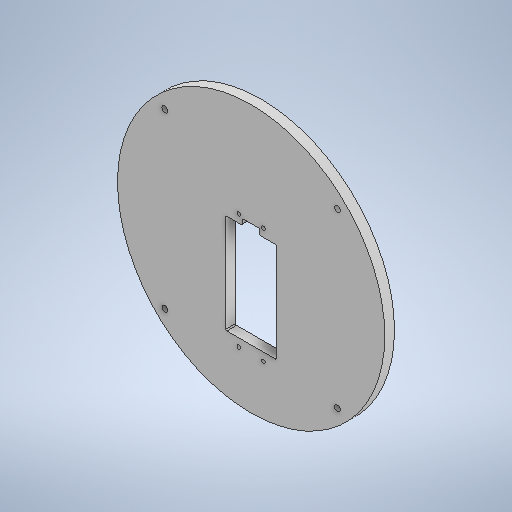
# Autodesk Inventor part: bottom-plate
Saved by Autodesk Inventor 2025 (Build 290162000, 162)
## iProperties
Created: 2024-05-28
Part Number: bottom-plate
Material: Generic
Document SubType Name: Modeling
Designer: hifzh
Density: 1 g/cm^3
Appearance: Default
Author: hifzh
## iProperties of the stored document bottom-plate_3DPrint.ipt
Created: 2024-07-12
Part Number: bottom-plate_3DPrint
Material: Generic
Document SubType Name: Modeling
Designer: hifzhil
Density: 1 g/cm^3
Appearance: Default
Author: hifzhil
Autodesk Inventor part; units mm, degrees
sketch "Sketch1" plane through (0, 0, 0) normal (0, 0, 1) x (1, 0, 0)
  circle A0 centre (0, 0) radius 55
  dimension "d0" = 110
  constraints: 1 centre point, 1 coincident
  measures "d0" diameter of A0
extrude "Extrusion1" add sketch "Sketch1" along normal blind 4
ref_plane "Work Plane1" through (0, 0, 4) normal (0, 0, 1) x (1, 0, 0)
sketch "Sketch2" plane through (0, 0, 4) normal (0, 0, 1) x (1, 0, 0)
  line L0 (-10.406, 10.152) -> (10.406, 10.152)
  line L1 (10.406, 10.152) -> (10.406, -30.726)
  line L2 (10.406, -30.726) -> (-10.406, -30.726)
  line L3 (-10.406, -30.726) -> (-10.406, 10.152)
  circle A0 centre (-35.532, 35.532) radius 1.5
  circle A1 centre (-35.532, -35.532) radius 1.5
  circle A2 centre (35.532, -35.532) radius 1.5
  circle A3 centre (35.532, 35.532) radius 1.5
  circle A4 centre (-5.08, 13.462) radius 1
  circle A5 centre (5.08, 13.462) radius 1
  circle A6 centre (-5.08, -34.036) radius 1
  circle A7 centre (5.08, -34.036) radius 1
  point P0 (0, 0)
  point P1 (0, 10.152)
  point P2 (0, -30.726)
  dimension "d78" = 30.226
  dimension "d80" = 5.08
  dimension "d82" = 5.08
  dimension "d4" = 20.812
  dimension "d5" = 40.878
  dimension "d6" = 10.152
  dimension "d7" = 3
  dimension "d8" = 3
  dimension "d9" = 3
  dimension "d10" = 3
  dimension "d11" = 2
  dimension "d12" = 2
  dimension "d13" = 2
  dimension "d14" = 2
  dimension "d15" = 35.532
  dimension "d16" = 35.532
  dimension "d17" = 35.532
  dimension "d18" = 35.532
  dimension "d19" = 35.532
  dimension "d20" = 35.532
  dimension "d21" = 35.532
  dimension "d22" = 35.532
  dimension "d23" = 10.16
  dimension "d24" = 10.16
  dimension "d25" = 3.31
  dimension "d26" = 3.31
  dimension "d27" = 3.31
  dimension "d28" = 3.31
  dimension "d47" = 30.726
  dimension "d48" = 5.08
  dimension "d49" = 5.08
  dimension "d50" = 5.08
  dimension "d51" = 5.08
  dimension "d137" = 10.152
  constraints: 8 centre point, 8 end point, 2 midpoint, 2 parallel, 1 horizontal, 1 perpendicular, 1 vertical alignment
  measures "d4" distance of L0.start L0.end
  measures "d5" distance of L0.end L1.end
  measures "d6" distance from line of point (0, 0) L0
  measures "d7" diameter of A0
  measures "d8" diameter of A1
  measures "d9" diameter of A2
  measures "d10" diameter of A3
  measures "d11" diameter of A4
  measures "d12" diameter of A5
  measures "d13" diameter of A6
  measures "d14" diameter of A7
  measures "d15" horizontal distance of point (0, 0) A0.centre
  measures "d16" horizontal distance of point (0, 0) A0.centre
  measures "d17" horizontal distance of point (0, 0) A3.centre
  measures "d18" horizontal distance of point (0, 0) A3.centre
  measures "d19" horizontal distance of point (0, 0) A2.centre
  measures "d20" horizontal distance of point (0, 0) A2.centre
  measures "d21" horizontal distance of point (0, 0) A1.centre
  measures "d22" horizontal distance of point (0, 0) A1.centre
  measures "d23" distance of A5.centre A4.centre
  measures "d24" distance of A7.centre A6.centre
  measures "d25" distance from line of L0 A4.centre
  measures "d26" distance from line of L0 A5.centre
  measures "d27" distance from line of L2 A6.centre
  measures "d28" distance from line of L2 A7.centre
  measures "d47" distance of point (0, -30.726) point (0, 0)
  measures "d48" horizontal distance of point (0, 0) A5.centre
  measures "d49" horizontal distance of point (0, 0) A4.centre
  measures "d50" horizontal distance of point (0, 0) A7.centre
  measures "d51" horizontal distance of point (0, 0) A6.centre
  measures "d137" distance of point (0, 10.152) point (0, 0)
extrude "Extrusion2" cut sketch "Sketch2" against normal blind 4 contours L0 L1 L2 L3
ref_plane "Work Plane2" through (0, 0, 4) normal (0, 0, 1) x (1, 0, 0)
sketch "Sketch3" plane through (0, 0, 4) normal (0, 0, 1) x (1, 0, 0)
  circle A0 centre (-35.577, 35.5342) radius 2.5
  circle A1 centre (-35.5225, -35.5931) radius 2.5
  circle A2 centre (35.5095, -35.5931) radius 2.5
  circle A3 centre (35.5095, 35.4262) radius 2.5
  point P0 (0, 0)
  constraints: 4 centre point
ref_plane "Work Plane3" through (0, 0, 0) normal (0, 0, 1) x (1, 0, 0)
sketch "Sketch4" plane through (0, 0, 0) normal (0, 0, 1) x (1, 0, 0)
  circle A0 centre (-35.577, 35.5342) radius 2.5
  circle A1 centre (-35.5225, -35.5931) radius 2.5
  circle A2 centre (35.5095, -35.5931) radius 2.5
  circle A3 centre (35.5095, 35.4262) radius 2.5
  point P0 (0, 0)
  point P1 (0, 0)
  dimension "d41" = 5
  dimension "d42" = 5
  dimension "d43" = 5
  dimension "d44" = 5
  constraints: 4 centre point
  measures "d41" diameter of A0
  measures "d42" diameter of A1
  measures "d43" diameter of A2
  measures "d44" diameter of A3
extrude "Extrusion3" cut sketch "Sketch4" along normal blind 0.657
ref_plane "Work Plane4" through (0, 0, 0) normal (0, 0, -1) x (-1, 0, 0)
sketch "Sketch5" plane through (0, 0, 0) normal (0, 0, -1) x (-1, 0, 0)
  line L0 (-9.906, 9.652) -> (9.906, 9.652)
  line L1 (9.906, 9.652) -> (9.906, -30.226)
  line L2 (9.906, -30.226) -> (-9.906, -30.226)
  line L3 (-9.906, -30.226) -> (-9.906, 9.652)
  circle A0 centre (-35.532, 35.532) radius 1.5
  circle A1 centre (-35.532, -35.532) radius 1.5
  circle A2 centre (35.532, -35.532) radius 1.5
  circle A3 centre (35.532, 35.532) radius 1.5
  circle A4 centre (-5.08, 13.462) radius 1
  circle A5 centre (5.08, 13.462) radius 1
  circle A6 centre (-5.08, -34.036) radius 1
  circle A7 centre (5.08, -34.036) radius 1
  point P0 (0, 0)
  point P1 (0, 0)
  point P2 (0, 9.652)
  point P3 (0, -30.226)
  dimension "d53" = 19.812
  dimension "d54" = 39.878
  dimension "d55" = 9.652
  dimension "d56" = 3
  dimension "d57" = 3
  dimension "d58" = 3
  dimension "d59" = 3
  dimension "d60" = 2
  dimension "d61" = 2
  dimension "d62" = 2
  dimension "d63" = 2
  dimension "d64" = 35.532
  dimension "d65" = 35.532
  dimension "d66" = 35.532
  dimension "d67" = 35.532
  dimension "d68" = 35.532
  dimension "d69" = 35.532
  dimension "d70" = 35.532
  dimension "d71" = 35.532
  dimension "d72" = 10.16
  dimension "d73" = 10.16
  dimension "d74" = 3.81
  dimension "d75" = 3.81
  dimension "d76" = 3.81
  dimension "d77" = 3.81
  dimension "d78" = 30.226
  dimension "d79" = 5.08
  dimension "d80" = 5.08
  dimension "d81" = 5.08
  dimension "d82" = 5.08
  constraints: 8 centre point, 8 end point, 2 midpoint, 2 parallel, 1 horizontal, 1 perpendicular, 1 vertical alignment
  measures "d53" distance of L0.start L0.end
  measures "d54" distance of L0.end L1.end
  measures "d55" distance from line of point (0, 0) L0
  measures "d56" diameter of A0
  measures "d57" diameter of A1
  measures "d58" diameter of A2
  measures "d59" diameter of A3
  measures "d60" diameter of A4
  measures "d61" diameter of A5
  measures "d62" diameter of A6
  measures "d63" diameter of A7
  measures "d64" horizontal distance of point (0, 0) A0.centre
  measures "d65" horizontal distance of point (0, 0) A0.centre
  measures "d66" horizontal distance of point (0, 0) A3.centre
  measures "d67" horizontal distance of point (0, 0) A3.centre
  measures "d68" horizontal distance of point (0, 0) A2.centre
  measures "d69" horizontal distance of point (0, 0) A2.centre
  measures "d70" horizontal distance of point (0, 0) A1.centre
  measures "d71" horizontal distance of point (0, 0) A1.centre
  measures "d72" distance of A5.centre A4.centre
  measures "d73" distance of A7.centre A6.centre
  measures "d74" distance from line of L0 A4.centre
  measures "d75" distance from line of L0 A5.centre
  measures "d76" distance from line of L2 A6.centre
  measures "d77" distance from line of L2 A7.centre
  measures "d78" distance of point (0, -30.226) point (0, 0)
  measures "d79" horizontal distance of point (0, 0) A5.centre
  measures "d80" horizontal distance of point (0, 0) A4.centre
  measures "d81" horizontal distance of point (0, 0) A7.centre
  measures "d82" horizontal distance of point (0, 0) A6.centre
hole "Hole1" at (35.532, 35.532, 0) at (-35.532, 35.532, 0) at (35.532, -35.532, 0) at (-35.532, -35.532, 0) direction (0, 0, 1) diameter 2.459 depth 4 tip angle 118 thread size "M3x0.5" class "6H" standard "ANSI Metric M Profile"
ref_plane "Work Plane5" through (0, 0, 0) normal (0, 0, -1) x (-1, 0, 0)
sketch "Sketch6" plane through (0, 0, 0) normal (0, 0, -1) x (-1, 0, 0)
  line L0 (-9.906, 9.652) -> (9.906, 9.652)
  line L1 (9.906, 9.652) -> (9.906, -30.226)
  line L2 (9.906, -30.226) -> (-9.906, -30.226)
  line L3 (-9.906, -30.226) -> (-9.906, 9.652)
  circle A0 centre (-35.532, 35.532) radius 1.5
  circle A1 centre (-35.532, -35.532) radius 1.5
  circle A2 centre (35.532, -35.532) radius 1.5
  circle A3 centre (35.532, 35.532) radius 1.5
  circle A4 centre (-5.08, 13.462) radius 1
  circle A5 centre (5.08, 13.462) radius 1
  circle A6 centre (-5.08, -34.036) radius 1
  circle A7 centre (5.08, -34.036) radius 1
  point P0 (0, 0)
  point P1 (0, 0)
  point P2 (0, 0)
  point P3 (0, 9.652)
  point P4 (0, -30.226)
  dimension "d91" = 19.812
  dimension "d92" = 39.878
  dimension "d93" = 9.652
  dimension "d94" = 3
  dimension "d95" = 3
  dimension "d96" = 3
  dimension "d97" = 3
  dimension "d98" = 2
  dimension "d99" = 2
  dimension "d100" = 2
  dimension "d101" = 2
  dimension "d102" = 35.532
  dimension "d103" = 35.532
  dimension "d104" = 35.532
  dimension "d105" = 35.532
  dimension "d106" = 35.532
  dimension "d107" = 35.532
  dimension "d108" = 35.532
  dimension "d109" = 35.532
  dimension "d110" = 10.16
  dimension "d111" = 10.16
  dimension "d112" = 3.81
  dimension "d113" = 3.81
  dimension "d114" = 3.81
  dimension "d115" = 3.81
  dimension "d116" = 30.226
  dimension "d117" = 5.08
  dimension "d118" = 5.08
  dimension "d119" = 5.08
  dimension "d120" = 5.08
  constraints: 8 centre point, 8 end point, 2 midpoint, 2 parallel, 1 horizontal, 1 perpendicular, 1 vertical alignment
  measures "d91" distance of L0.start L0.end
  measures "d92" distance of L0.end L1.end
  measures "d93" distance from line of point (0, 0) L0
  measures "d94" diameter of A0
  measures "d95" diameter of A1
  measures "d96" diameter of A2
  measures "d97" diameter of A3
  measures "d98" diameter of A4
  measures "d99" diameter of A5
  measures "d100" diameter of A6
  measures "d101" diameter of A7
  measures "d102" horizontal distance of point (0, 0) A0.centre
  measures "d103" horizontal distance of point (0, 0) A0.centre
  measures "d104" horizontal distance of point (0, 0) A3.centre
  measures "d105" horizontal distance of point (0, 0) A3.centre
  measures "d106" horizontal distance of point (0, 0) A2.centre
  measures "d107" horizontal distance of point (0, 0) A2.centre
  measures "d108" horizontal distance of point (0, 0) A1.centre
  measures "d109" horizontal distance of point (0, 0) A1.centre
  measures "d110" distance of A5.centre A4.centre
  measures "d111" distance of A7.centre A6.centre
  measures "d112" distance from line of L0 A4.centre
  measures "d113" distance from line of L0 A5.centre
  measures "d114" distance from line of L2 A6.centre
  measures "d115" distance from line of L2 A7.centre
  measures "d116" distance of point (0, -30.226) point (0, 0)
  measures "d117" horizontal distance of point (0, 0) A5.centre
  measures "d118" horizontal distance of point (0, 0) A4.centre
  measures "d119" horizontal distance of point (0, 0) A7.centre
  measures "d120" horizontal distance of point (0, 0) A6.centre
hole "Hole2" at (-5.08, 13.462, 0) at (5.08, 13.462, 0) at (-5.08, -34.036, 0) at (5.08, -34.036, 0) direction (0, 0, 1) diameter 1.567 depth 4 tip angle 118 thread size "M2x0.4" class "6H" standard "ANSI Metric M Profile"
fillet "Fillet1" radius 0.4125 4 edges at (10.406, -30.726, 2) (-10.406, -30.726, 2) (10.406, 10.152, 2) (-10.406, 10.152, 2)
ref_plane "Work Plane6" through (0, 0, 0) normal (0, 0, -1) x (-1, 0, 0)
sketch "Sketch7" plane through (0, 0, 0) normal (0, 0, -1) x (-1, 0, 0)
  line L0 (3.5, 12.552) -> (-3.5, 12.552)
  line L1 (-3.5, 12.552) -> (-3.5, 10.052)
  line L2 (-3.5, 10.052) -> (3.5, 10.052)
  line L3 (3.5, 10.052) -> (3.5, 12.552)
  line L4 (-9.9935, 10.152) -> (9.9935, 10.152) projected
  point P0 (0, 0)
  point P1 (-3.5, 10.152)
  point P2 (3.5, 10.152)
  dimension "d130" = 2.5
  dimension "d131" = 7
  dimension "d132" = 0.1
  dimension "d133" = 3.5
  constraints: 8 end point, 2 parallel, 1 horizontal, 1 perpendicular
  measures "d130" distance of L2.end L0.start
  measures "d131" distance of L0.start L0.end
  measures "d132" distance between parallel lines of L4 L2
  measures "d133" distance from line of point (0, 0) L3
extrude "Extrusion4" cut sketch "Sketch7" against normal blind 4 contours L3 L4 L1 L0
fillet "Fillet2" radius 0.5 4 edges at (-3.5, 12.552, 2) (-3.5, 10.152, 2) (3.5, 12.552, 2) (3.5, 10.152, 2)
body "Solid1"
